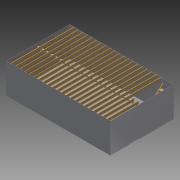
# Autodesk Inventor part: Vetturi_Flat Ceiling
Saved by Autodesk Inventor 2013 SP2 (Build 170200200, 200)
## iProperties
Created: 2010-06-22
Part Number: Vetturi_Flat Ceiling
Document SubType Name: Modeling
Designer: taylorm
Density: 1 g/cm^3
Material: Generic
Author: taylorm
Autodesk Inventor part; units mm, degrees
sketch "Sketch2" plane through (0, 0, 0) normal (0, 1, 0) x (-1, 0, 0)
  line L0 (-0.9786, 3723.3655) -> (9199.0214, 3723.3655)
  line L1 (9199.0214, 3723.3655) -> (9199.0214, -1876.6345)
  line L2 (9199.0214, -1876.6345) -> (-0.9786, -1876.6345)
  line L3 (-0.9786, -1876.6345) -> (-0.9786, 3723.3655)
  point P0 (0, 0)
  dimension "d0" = 9200
  dimension "d1" = 5600
  constraints: 8 end point, 2 parallel, 1 horizontal, 1 perpendicular
  measures "d0" distance between parallel lines of L3 L1
  measures "d1" distance between parallel lines of L0 L2
ref_plane "Work Plane1" through (0.9786, 0, 3723.3655) normal (0, 0, 1) x (1, 0, 0)
sketch "Sketch3" plane through (0.9786, 0, 3723.3655) normal (0, 0, 1) x (1, 0, 0)
  line L0 (0, 0) -> (-9200, 0) projected
  line L1 (-9200, 0) -> (-9200, 2640)
  line L2 (-9200, 2640) -> (0, 2640)
  line L3 (0, 2640) -> (0, 0)
  point P0 (-0.9786, 0)
  dimension "d2" = 2640
  constraints: 6 end point, 3 perpendicular
  measures "d2" distance between parallel lines of L0 L2
ref_plane "Work Plane2" through (0.9786, 0, -1876.6345) normal (0, 0, 1) x (1, 0, 0)
sketch "Sketch4" plane through (0.9786, 0, -1876.6345) normal (0, 0, 1) x (1, 0, 0)
  line L0 (-9200, 0) -> (0, 0) projected
  line L1 (-9200, 0) -> (-9200, 2640)
  line L2 (-9200, 2640) -> (0, 2640)
  line L3 (0, 2640) -> (0, 0)
  point P0 (-0.9786, 0)
  dimension "d3" = 2640
  constraints: 6 end point, 2 perpendicular, 1 parallel
  measures "d3" distance between parallel lines of L0 L2
ref_plane "Work Plane3" through (0.9786, 0, 3723.3655) normal (-1, 0, 0) x (0, 1, 0)
sketch "Sketch5" plane through (0.9786, 0, 3723.3655) normal (-1, 0, 0) x (0, 1, 0)
  line L0 (3168, 0) -> (-528, 0) projected
  line L1 (3168, 5600) -> (-528, 5600) projected
  line L2 (2640, 0) -> (0, 0) projected
  line L3 (0, 5600) -> (0, 0) projected
  line L4 (2640, 5600) -> (0, 5600) projected
  line L5 (2640, 0) -> (2640, 5600)
  line L6 (2640, 5600) -> (0, 5600)
  line L7 (0, 5600) -> (0, 0)
  line L8 (0, 0) -> (2640, 0)
  line L9 (0, 1600) -> (2125, 1600)
  line L10 (2125, 1600) -> (2125, 2510)
  line L11 (2125, 2510) -> (0, 2510)
  line L12 (0, 2510) -> (0, 5600)
  line L13 (0, 5600) -> (2640, 5600)
  line L14 (2640, 5600) -> (2640, 0)
  line L15 (2640, 0) -> (0, 0)
  line L16 (0, 0) -> (0, 1600)
  point P0 (0, 3723.3655)
  dimension "d60" = 1600
  dimension "d61" = 910
  dimension "d62" = 2125
  constraints: 24 end point, 9 perpendicular, 2 collinear, 2 point on line, 1 parallel
  measures "d60" distance between parallel lines of L9 L15
  measures "d61" distance between parallel lines of L11 L9
  measures "d62" distance between parallel lines of L3 L10
ref_plane "Work Plane4" through (-9199.0214, 0, 3723.3655) normal (-1, 0, 0) x (0, 1, 0)
sketch "Sketch6" plane through (-9199.0214, 0, 3723.3655) normal (-1, 0, 0) x (0, 1, 0)
  line L0 (0, 0) -> (0, 5600) projected
  line L1 (0, 0) -> (2640, 0) projected
  line L2 (0, 5600) -> (2640, 5600) projected
  line L3 (0, 0) -> (0, 5600)
  line L4 (0, 5600) -> (2640, 5600)
  line L5 (2640, 5600) -> (2640, 0)
  line L6 (2640, 0) -> (0, 0)
  point P0 (0, 3723.3655)
  constraints: 8 end point, 3 perpendicular, 1 collinear
ref_plane "Work Plane5" through (-9199.0214, 2640, 3723.3655) normal (0, 1, 0) x (1, 0, 0)
sketch "Sketch7" plane through (-9199.0214, 2640, 3723.3655) normal (0, 1, 0) x (1, 0, 0)
  line L0 (0, 0) -> (9200, 0) projected
  line L1 (0, 5600) -> (0, 0) projected
  line L2 (0, 5600) -> (9200, 5600) projected
  line L3 (9200, 0) -> (9200, 5600) projected
  line L4 (0, 0) -> (9200, 0)
  line L5 (9200, 0) -> (9200, 5600)
  line L6 (9200, 5600) -> (0, 5600)
  line L7 (0, 5600) -> (0, 0)
  line L8 (8300, 5600) -> (8300, 2900)
  line L9 (8300, 2900) -> (9200, 2900)
  line L10 (9200, 5600) -> (8300, 5600)
  line L11 (0, 5600) -> (8300, 5600)
  line L12 (8300, 5600) -> (8300, 2900)
  line L13 (8300, 2900) -> (9200, 2900)
  line L14 (9200, 2900) -> (9200, 0)
  line L15 (9200, 0) -> (0, 0)
  line L16 (0, 0) -> (0, 5600)
  point P0 (9199.0214, 3723.3655)
  dimension "d4" = 900
  dimension "d5" = 2700
  constraints: 26 end point, 9 perpendicular, 3 collinear, 2 point on line, 1 parallel
  measures "d4" distance of L9.end L8.end
  measures "d5" distance between parallel lines of L2 L9
extrude "Extrusion1" [suppressed]
sketch "Sketch8" plane through (-9199.0214, 2640, 3723.3655) normal (0, 1, 0) x (1, 0, 0)
  line L0 (0, 0) -> (9200, 0) projected
  line L1 (0, 5600) -> (0, 0) projected
  line L2 (8300, 5600) -> (0, 5600) projected
  line L3 (8300, 2900) -> (8300, 5600) projected
  line L4 (9200, 2900) -> (8300, 2900) projected
  line L5 (9200, 0) -> (9200, 5600) projected
  line L6 (0, 5600) -> (9200, 5600) projected
  line L7 (368, 0) -> (368, 5600)
  line L8 (368, 5600) -> (404.8, 5600)
  line L9 (404.8, 5600) -> (404.8, 0)
  line L10 (404.8, 0) -> (368, 0)
  line L11 (772.8, 0) -> (772.8, 5600)
  line L12 (772.8, 5600) -> (809.6, 5600)
  line L13 (809.6, 5600) -> (809.6, 0)
  line L14 (809.6, 0) -> (772.8, 0)
  line L15 (1177.6, 0) -> (1177.6, 5600)
  line L16 (1177.6, 5600) -> (1214.4, 5600)
  line L17 (1214.4, 5600) -> (1214.4, 0)
  line L18 (1214.4, 0) -> (1177.6, 0)
  line L19 (1582.4, 0) -> (1582.4, 5600)
  line L20 (1582.4, 5600) -> (1619.2, 5600)
  line L21 (1619.2, 5600) -> (1619.2, 0)
  line L22 (1619.2, 0) -> (1582.4, 0)
  line L23 (1987.2, 5600) -> (1987.2, 0)
  line L24 (1987.2, 0) -> (2024, 0)
  line L25 (2024, 0) -> (2024, 5600)
  line L26 (2024, 5600) -> (1987.2, 5600)
  line L27 (2392, 5600) -> (2392, 0)
  line L28 (2392, 0) -> (2428.8, 0)
  line L29 (2428.8, 0) -> (2428.8, 5600)
  line L30 (2392, 5600) -> (2428.8, 5600)
  line L31 (2796.8, 5600) -> (2796.8, 0)
  line L32 (2796.8, 0) -> (2833.6, 0)
  line L33 (2833.6, 0) -> (2796.8, 0)
  line L34 (2833.6, 0) -> (2833.6, 5600)
  line L35 (2833.6, 5600) -> (2796.8, 5600)
  line L36 (3201.6, 5600) -> (3201.6, 0)
  line L37 (3201.6, 0) -> (3238.4, 0)
  line L38 (3238.4, 0) -> (3238.4, 5600)
  line L39 (3238.4, 5600) -> (3201.6, 5600)
  line L40 (3606.4, 5600) -> (3606.4, 0)
  line L41 (3606.4, 0) -> (3643.2, 0)
  line L42 (3643.2, 0) -> (3643.2, 5600)
  line L43 (3643.2, 5600) -> (3606.4, 5600)
  line L44 (4011.2, 5600) -> (4011.2, 0)
  line L45 (4011.2, 0) -> (4048, 0)
  line L46 (4048, 0) -> (4048, 5600)
  line L47 (4048, 5600) -> (4011.2, 5600)
  line L48 (4416, 5600) -> (4416, 0)
  line L49 (4416, 0) -> (4452.8, 0)
  line L50 (4452.8, 0) -> (4452.8, 5600)
  line L51 (4416, 5600) -> (4452.8, 5600)
  line L52 (4820.8, 5600) -> (4820.8, 0)
  line L53 (4820.8, 0) -> (4857.6, 0)
  line L54 (4857.6, 0) -> (4857.6, 5600)
  line L55 (4857.6, 5600) -> (4820.8, 5600)
  line L56 (5225.6, 5600) -> (5225.6, 0)
  line L57 (5225.6, 0) -> (5262.4, 0)
  line L58 (5262.4, 0) -> (5262.4, 5600)
  line L59 (5262.4, 5600) -> (5225.6, 5600)
  line L60 (5630.4, 5600) -> (5630.4, 0)
  line L61 (5630.4, 0) -> (5667.2, 0)
  line L62 (5667.2, 0) -> (5667.2, 5600)
  line L63 (5667.2, 5600) -> (5630.4, 5600)
  line L64 (6035.2, 5600) -> (6035.2, 0)
  line L65 (6035.2, 0) -> (6072, 0)
  line L66 (6072, 0) -> (6072, 5600)
  line L67 (6072, 5600) -> (6035.2, 5600)
  line L68 (6440, 5600) -> (6440, 0)
  line L69 (6440, 0) -> (6476.8, 0)
  line L70 (6476.8, 0) -> (6476.8, 5600)
  line L71 (6476.8, 5600) -> (6440, 5600)
  line L72 (6844.8, 5600) -> (6844.8, 0)
  line L73 (6844.8, 0) -> (6881.6, 0)
  line L74 (6881.6, 0) -> (6881.6, 5600)
  line L75 (6881.6, 5600) -> (6844.8, 5600)
  line L76 (7249.6, 5600) -> (7249.6, 0)
  line L77 (7249.6, 0) -> (7286.4, 0)
  line L78 (7286.4, 0) -> (7286.4, 5600)
  line L79 (7286.4, 5600) -> (7249.6, 5600)
  line L80 (7654.4, 5600) -> (7654.4, 0)
  line L81 (7654.4, 0) -> (7691.2, 0)
  line L82 (7691.2, 0) -> (7691.2, 5600)
  line L83 (7691.2, 5600) -> (7654.4, 5600)
  line L84 (8059.2, 5600) -> (8059.2, 0)
  line L85 (8059.2, 0) -> (8096, 0)
  line L86 (8096, 0) -> (8096, 5600)
  line L87 (8059.2, 5600) -> (8096, 5600)
  line L88 (8464, 0) -> (8464, 2800)
  line L89 (8464, 2800) -> (8500.8, 2800)
  line L90 (8500.8, 2800) -> (8500.8, 0)
  line L91 (8464, 0) -> (8500.8, 0)
  line L92 (8868.8, 0) -> (8868.8, 2800)
  line L93 (8868.8, 2800) -> (8905.6, 2800)
  line L94 (8905.6, 2800) -> (8905.6, 0)
  line L95 (8868.8, 0) -> (8905.6, 0)
  point P0 (9199.0214, 3723.3655)
  dimension "d8" = 368
  dimension "d9" = 404.8
  dimension "d10" = 772.8
  dimension "d11" = 809.6
  dimension "d12" = 1177.6
  dimension "d13" = 1214.4
  dimension "d14" = 1582.4
  dimension "d15" = 1619.2
  dimension "d16" = 1987.2
  dimension "d17" = 2024
  dimension "d18" = 2392
  dimension "d19" = 2428.8
  dimension "d20" = 2796.8
  dimension "d21" = 2833.6
  dimension "d22" = 3201.6
  dimension "d23" = 3238.4
  dimension "d24" = 3606.4
  dimension "d25" = 3643.2
  dimension "d26" = 4011.2
  dimension "d27" = 4048
  dimension "d28" = 4416
  dimension "d29" = 4452.8
  dimension "d30" = 4820.8
  dimension "d31" = 4857.6
  dimension "d32" = 5225.6
  dimension "d33" = 5262.4
  dimension "d34" = 5630.4
  dimension "d35" = 5667.2
  dimension "d36" = 6035.2
  dimension "d37" = 6072
  dimension "d38" = 6440
  dimension "d39" = 6476.8
  dimension "d40" = 6844.8
  dimension "d41" = 6881.6
  dimension "d42" = 7249.6
  dimension "d43" = 7286.4
  dimension "d44" = 7654.4
  dimension "d45" = 7691.2
  dimension "d46" = 8059.2
  dimension "d47" = 8096
  dimension "d48" = 8464
  dimension "d49" = 8500.8
  dimension "d50" = 2800
  dimension "d51" = 2800
  dimension "d52" = 8868.8
  dimension "d53" = 8905.6
  constraints: 178 end point, 35 perpendicular, 23 vertical, 6 collinear, 3 horizontal, 2 parallel, 86 other
  measures "d8" distance between parallel lines of L7 L1
  measures "d9" distance between parallel lines of L9 L1
  measures "d10" distance between parallel lines of L11 L1
  measures "d11" distance between parallel lines of L13 L1
  measures "d12" distance between parallel lines of L15 L1
  measures "d13" distance between parallel lines of L1 L17
  measures "d14" distance between parallel lines of L19 L1
  measures "d15" distance between parallel lines of L21 L1
  measures "d16" distance between parallel lines of L1 L23
  measures "d17" distance between parallel lines of L25 L1
  measures "d18" distance between parallel lines of L27 L1
  measures "d19" distance between parallel lines of L29 L1
  measures "d20" distance between parallel lines of L31 L1
  measures "d21" distance between parallel lines of L34 L1
  measures "d22" distance between parallel lines of L36 L1
  measures "d23" distance between parallel lines of L38 L1
  measures "d24" distance between parallel lines of L40 L1
  measures "d25" distance between parallel lines of L42 L1
  measures "d26" distance between parallel lines of L44 L1
  measures "d27" distance between parallel lines of L46 L1
  measures "d28" distance between parallel lines of L48 L1
  measures "d29" distance between parallel lines of L50 L1
  measures "d30" distance between parallel lines of L52 L1
  measures "d31" distance between parallel lines of L54 L1
  measures "d32" distance between parallel lines of L56 L1
  measures "d33" distance between parallel lines of L58 L1
  measures "d34" distance between parallel lines of L60 L1
  measures "d35" distance between parallel lines of L62 L1
  measures "d36" distance between parallel lines of L64 L1
  measures "d37" distance between parallel lines of L66 L1
  measures "d38" distance between parallel lines of L68 L1
  measures "d39" distance between parallel lines of L70 L1
  measures "d40" distance between parallel lines of L72 L1
  measures "d41" distance between parallel lines of L74 L1
  measures "d42" distance between parallel lines of L76 L1
  measures "d43" distance between parallel lines of L78 L1
  measures "d44" distance between parallel lines of L80 L1
  measures "d45" distance between parallel lines of L82 L1
  measures "d46" distance between parallel lines of L84 L1
  measures "d47" distance between parallel lines of L86 L1
  measures "d48" distance between parallel lines of L88 L1
  measures "d49" distance between parallel lines of L90 L1
  measures "d50" distance of the line from the sketch origin of L89
  measures "d51" distance of the line from the sketch origin of L93
  measures "d52" distance between parallel lines of L92 L1
  measures "d53" distance between parallel lines of L1 L94
extrude "Extrusion2" add sketch "Sketch8" against normal blind 240 contours L7 L2 L9 L0 | L11 L2 L13 L0 | L15 L2 L17 L0 | L19 L2 L21 L0 | L23 L2 L25 L0 | L27 L2 L29 L0 | L31 L2 L34 L0 | L36 L2 L38 L0 | L40 L2 L42 L0 | L44 L2 L46 L0 | L48 L2 L50 L0 | L52 L2 L54 L0 | L56 L2 L58 L0 | L60 L2 L62 L0 | L64 L2 L66 L0 | L68 L2 L70 L0 | L72 L2 L74 L0 | L76 L2 L78 L0 | L80 L2 L82 L0 | L84 L2 L86 L0 | L88 L89 L90 L0 | L92 L93 L94 L0
ref_plane "Work Plane7" through (-293.4214, 2400, 3723.3655) normal (0, 1, 0) x (-1, 0, 0)
sketch "Sketch9" plane through (-293.4214, 2400, 3723.3655) normal (0, 1, 0) x (-1, 0, 0)
  line L0 (-294.4, 0) -> (-294.4, -5600) projected
  line L1 (8905.6, 0) -> (-294.4, 0) projected
  line L2 (8905.6, -5600) -> (-294.4, -5600) projected
  line L3 (8905.6, -5600) -> (8905.6, 0) projected
  line L4 (-294.4, -2720) -> (8905.6, -2720)
  line L5 (8905.6, -2720) -> (8905.6, -2800)
  line L6 (8905.6, -2800) -> (-294.4, -2800)
  line L7 (-294.4, -2800) -> (-294.4, -2720)
  point P0 (-293.4214, -3723.3655)
  dimension "d56" = 2720
  dimension "d57" = 2800
  constraints: 8 end point, 3 perpendicular, 2 midpoint, 2 point on line
  measures "d56" distance between parallel lines of L4 L1
  measures "d57" distance between parallel lines of L6 L1
extrude "Extrusion3" add sketch "Sketch9" against normal blind 180 contours L4 L3 L6 L0
extrude "Extrusion4" add sketch "Sketch5" along normal blind 12.7 contours L0 L3 L9 L10 L11 L1 L5
sketch "Sketch10" plane through (0.9786, 0, 3723.3655) normal (-1, 0, 0) x (0, 1, 0)
  line L0 (2125, 2510) -> (2125, 1600) projected
  line L1 (2125, 1600) -> (0, 1600) projected
  line L2 (0, 2510) -> (2125, 2510) projected
  line L3 (2125, 1600) -> (2125, 2510)
  line L4 (2125, 2510) -> (25, 2510)
  line L5 (25, 2510) -> (25, 1600)
  line L6 (25, 1600) -> (2125, 1600)
  point P0 (0, 3723.3655)
  dimension "d65" = 2100
  constraints: 8 end point, 2 perpendicular, 2 point on line, 1 collinear
  measures "d65" distance between parallel lines of L5 L3
extrude "Extrusion5" add sketch "Sketch10" along normal blind 38.1
extrude "Extrusion6" add sketch "Sketch6" against normal blind 12.7
extrude "Extrusion7" add sketch "Sketch4" along normal blind 12.7
extrude "Extrusion8" add sketch "Sketch2" against normal blind 12.7
sketch "Sketch11" plane through (0.9786, 0, 3723.3655) normal (-1, 0, 0) x (0, 1, 0)
  line L0 (2627.3, 2900) -> (2627.3, 5600) projected
  line L1 (137.3, 3050.1877) -> (187.3, 3050.1877)
  line L2 (187.3, 3050.1877) -> (187.3, 3286.1877)
  line L3 (187.3, 3286.1877) -> (137.3, 3286.1877)
  line L4 (137.3, 3286.1877) -> (137.3, 3050.1877)
  line L5 (337.3, 3286.1877) -> (387.3, 3286.1877)
  line L6 (387.3, 3286.1877) -> (387.3, 3522.1877)
  line L7 (387.3, 3522.1877) -> (337.3, 3522.1877)
  line L8 (337.3, 3522.1877) -> (337.3, 3286.1877)
  line L9 (587.3, 3522.1877) -> (537.3, 3522.1877)
  line L10 (537.3, 3522.1877) -> (537.3, 3758.1877)
  line L11 (537.3, 3758.1877) -> (587.3, 3758.1877)
  line L12 (587.3, 3758.1877) -> (587.3, 3522.1877)
  line L13 (787.3, 3758.1877) -> (737.3, 3758.1877)
  line L14 (737.3, 3758.1877) -> (737.3, 3994.1877)
  line L15 (737.3, 3994.1877) -> (787.3, 3994.1877)
  line L16 (787.3, 3994.1877) -> (787.3, 3758.1877)
  line L17 (987.3, 3994.1877) -> (937.3, 3994.1877)
  line L18 (937.3, 3994.1877) -> (937.3, 4230.1877)
  line L19 (937.3, 4230.1877) -> (987.3, 4230.1877)
  line L20 (987.3, 4230.1877) -> (987.3, 3994.1877)
  line L21 (1187.3, 4230.1877) -> (1137.3, 4230.1877)
  line L22 (1137.3, 4230.1877) -> (1137.3, 4466.1877)
  line L23 (1137.3, 4466.1877) -> (1187.3, 4466.1877)
  line L24 (1187.3, 4466.1877) -> (1187.3, 4230.1877)
  line L25 (-12.7, 0) -> (-12.7, 5600) projected
  line L26 (1387.3, 4466.1877) -> (1337.3, 4466.1877)
  line L27 (1337.3, 4466.1877) -> (1337.3, 4702.1877)
  line L28 (1337.3, 4702.1877) -> (1387.3, 4702.1877)
  line L29 (1387.3, 4702.1877) -> (1387.3, 4466.1877)
  line L30 (1587.3, 4702.1877) -> (1537.3, 4702.1877)
  line L31 (1537.3, 4702.1877) -> (1537.3, 4938.1877)
  line L32 (1537.3, 4938.1877) -> (1587.3, 4938.1877)
  line L33 (1587.3, 4938.1877) -> (1587.3, 4702.1877)
  line L34 (1787.3, 4938.1877) -> (1737.3, 4938.1877)
  line L35 (1737.3, 4938.1877) -> (1737.3, 5174.1877)
  line L36 (1737.3, 5174.1877) -> (1787.3, 5174.1877)
  line L37 (1787.3, 5174.1877) -> (1787.3, 4938.1877)
  line L38 (1987.3, 5174.1877) -> (1937.3, 5174.1877)
  line L39 (1937.3, 5174.1877) -> (1937.3, 5410.1877)
  line L40 (1937.3, 5410.1877) -> (1987.3, 5410.1877)
  line L41 (1987.3, 5410.1877) -> (1987.3, 5174.1877)
  point P0 (0, 3723.3655)
  dimension "d74" = 200
  dimension "d75" = 236
  dimension "d76" = 600
  dimension "d77" = 400
  dimension "d78" = 800
  dimension "d79" = 1000
  dimension "d80" = 1200
  dimension "d81" = 50
  dimension "d82" = 50
  dimension "d83" = 50
  dimension "d84" = 50
  dimension "d85" = 50
  dimension "d86" = 50
  dimension "d87" = 236
  dimension "d88" = 236
  dimension "d89" = 236
  dimension "d90" = 236
  dimension "d91" = 236
  dimension "d92" = 236
  dimension "d93" = 236
  dimension "d94" = 236
  dimension "d95" = 236
  dimension "d96" = 236
  dimension "d97" = 50
  dimension "d98" = 50
  dimension "d99" = 50
  dimension "d100" = 50
  dimension "d101" = 236
  dimension "d102" = 200
  dimension "d103" = 200
  dimension "d104" = 200
  dimension "d105" = 200
  constraints: 80 end point, 20 parallel, 11 perpendicular, 9 collinear, 9 horizontal
  measures "d74" distance between parallel lines of L25 L2
  measures "d75" distance of L5.end L6.end
  measures "d76" distance between parallel lines of L25 L12
  measures "d77" distance between parallel lines of L25 L6
  measures "d78" distance between parallel lines of L25 L16
  measures "d79" distance between parallel lines of L25 L20
  measures "d80" distance between parallel lines of L25 L24
  measures "d81" distance between parallel lines of L4 L2
  measures "d82" distance between parallel lines of L8 L6
  measures "d83" distance between parallel lines of L10 L12
  measures "d84" distance between parallel lines of L14 L16
  measures "d85" distance between parallel lines of L18 L20
  measures "d86" distance between parallel lines of L22 L24
  measures "d87" distance between parallel lines of L3 L1
  measures "d88" distance between parallel lines of L7 L5
  measures "d89" distance between parallel lines of L11 L9
  measures "d90" distance between parallel lines of L15 L13
  measures "d91" distance between parallel lines of L23 L21
  measures "d92" distance of L19.end L17.start
  measures "d93" distance between parallel lines of L28 L26
  measures "d94" distance between parallel lines of L32 L30
  measures "d95" distance between parallel lines of L36 L34
  measures "d96" distance between parallel lines of L40 L38
  measures "d97" distance between parallel lines of L27 L29
  measures "d98" distance between parallel lines of L31 L33
  measures "d99" distance between parallel lines of L35 L37
  measures "d100" distance between parallel lines of L39 L41
  measures "d101" distance of L26.end L27.end
  measures "d102" distance between parallel lines of L24 L29
  measures "d103" distance between parallel lines of L29 L33
  measures "d104" distance between parallel lines of L33 L37
  measures "d105" distance between parallel lines of L37 L41
extrude "Extrusion9" add sketch "Sketch11" along normal blind 900
ref_plane "Work Plane8" through (-899.0214, 1987.3, -1686.8222) normal (1, 0, 0) x (0, 0, 1)
sketch "Sketch12" plane through (-899.0214, 1987.3, -1686.8222) normal (1, 0, 0) x (0, 0, 1)
  line L0 (-189.8123, 2000) -> (5410.1877, 2000) projected
  line L1 (-189.8123, -652.7) -> (5410.1877, -652.7) projected
  line L2 (-175.4791, -301.528) -> (2523.6937, 2000)
  line L3 (2523.6937, 2000) -> (2369.5704, 2000)
  line L4 (2369.5704, 2000) -> (-175.4791, -170.1103)
  line L5 (-175.4791, -301.528) -> (-175.4791, -170.1103)
  point P0 (1686.8222, 1987.3)
  dimension "d108" = 100
  constraints: 8 end point, 2 point on line, 1 parallel, 1 perpendicular
  measures "d108" distance between parallel lines of L4 L2
extrude "Extrusion10" add sketch "Sketch12" against normal blind 50
sketch "Sketch13" plane through (0, 0, 0) normal (0, 1, 0) x (-1, 0, 0)
  line L0 (-0.9786, 3723.3655) -> (9199.0214, 3723.3655) projected
  line L1 (9199.0214, 3723.3655) -> (9199.0214, -1863.9345) projected
  line L2 (9199.0214, 3723.3655) -> (8499.0214, 3723.3655)
  line L3 (8499.0214, 3723.3655) -> (8499.0214, 2723.3655)
  line L4 (8499.0214, 2723.3655) -> (9199.0214, 2723.3655)
  line L5 (9199.0214, 2723.3655) -> (9199.0214, 3723.3655)
  line L6 (6158.3377, 3723.3655) -> (5458.3377, 3723.3655)
  line L7 (5458.3377, 3723.3655) -> (5458.3377, 2723.3655)
  line L8 (5458.3377, 2723.3655) -> (6158.3377, 2723.3655)
  line L9 (6158.3377, 2723.3655) -> (6158.3377, 3723.3655)
  line L10 (5458.3377, 2723.3655) -> (6158.3377, 2723.3655)
  line L11 (6158.3377, 2723.3655) -> (6158.3377, 1723.3655)
  line L12 (6158.3377, 1723.3655) -> (5458.3377, 1723.3655)
  line L13 (5458.3377, 1723.3655) -> (5458.3377, 2723.3655)
  point P0 (0, 0)
  point P1 (9199.0214, -1876.6345)
  dimension "d111" = 700
  dimension "d112" = 1000
  dimension "d113" = 1000
  dimension "d114" = 1000
  dimension "d115" = 700
  dimension "d116" = 700
  constraints: 24 end point, 6 parallel, 3 horizontal, 3 perpendicular, 1 point on line
  measures "d111" distance between parallel lines of L5 L3
  measures "d112" distance between parallel lines of L0 L4
  measures "d113" distance between parallel lines of L0 L8
  measures "d114" distance between parallel lines of L12 L8
  measures "d115" distance between parallel lines of L7 L9
  measures "d116" distance between parallel lines of L13 L11
extrude "Extrusion11" add sketch "Sketch13" along normal blind 300 contours L0 L1 L4 L3
sketch "Sketch14" plane through (0, 0, 0) normal (0, 1, 0) x (-1, 0, 0)
  line L0 (-0.9786, 3723.3655) -> (9199.0214, 3723.3655) projected
  line L1 (9199.0214, 2723.3655) -> (9199.0214, -1863.9345) projected
  line L2 (4599.0214, 3723.3655) -> (3899.0214, 3723.3655)
  line L3 (3899.0214, 3723.3655) -> (3899.0214, 2723.3655)
  line L4 (3899.0214, 2723.3655) -> (4599.0214, 2723.3655)
  line L5 (4599.0214, 2723.3655) -> (4599.0214, 3723.3655)
  point P0 (0, 0)
  point P1 (9199.0214, -1876.6345)
  dimension "d119" = 4600
  dimension "d120" = 700
  dimension "d121" = 1000
  constraints: 8 end point, 2 parallel, 1 horizontal, 1 midpoint, 1 perpendicular
  measures "d119" distance between parallel lines of L1 L5
  measures "d120" distance between parallel lines of L5 L3
  measures "d121" distance between parallel lines of L0 L4
extrude "Extrusion12" add sketch "Sketch14" along normal blind 300
sketch "Sketch15" plane through (0, 0, 0) normal (0, 1, 0) x (-1, 0, 0)
  line L0 (9199.0214, 2723.3655) -> (9199.0214, -1863.9345) projected
  line L1 (4599.0214, 2723.3655) -> (3899.0214, 2723.3655) projected
  line L2 (3899.0214, 2723.3655) -> (4599.0214, 2723.3655)
  line L3 (4599.0214, 2723.3655) -> (4599.0214, 1723.3655)
  line L4 (4599.0214, 1723.3655) -> (3899.0214, 1723.3655)
  line L5 (3899.0214, 1723.3655) -> (3899.0214, 2723.3655)
  point P0 (0, 0)
  point P1 (9199.0214, -1876.6345)
  dimension "d124" = 700
  dimension "d125" = 1000
  constraints: 8 end point, 2 parallel, 1 horizontal, 1 perpendicular
  measures "d124" distance between parallel lines of L5 L3
  measures "d125" distance between parallel lines of L1 L4
extrude "Extrusion13" add sketch "Sketch15" along normal blind 300 separate body
extrude "Extrusion14" add sketch "Sketch3" along normal blind 12.7 separate body
body "Solid1"
body "Solid2"
body "Solid3"
